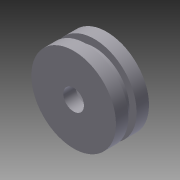
# Autodesk Inventor part: TU-005
Saved by Autodesk Inventor 2011 (Build 150229000, 229)
## iProperties
Created: 2008-06-13
Part Number: TU-005
Document SubType Name: Modeling
Designer: PN
Density: 2.71 g/cm^3
Material: Aluminum-6061
Description: Piston
Mass: 37.1113 g
Surface Area: 62.8633 cm^2
Volume: 13.6942 cm^3
Author: PN
Autodesk Inventor part; units mm, degrees
ref_plane "YZ Plane" through (0, 0, 0) normal (1, 0, 0) x (0, 1, 0)
ref_plane "XZ Plane" through (0, 0, 0) normal (0, 1, 0) x (-1, 0, 0)
ref_plane "XY Plane" through (0, 0, 0) normal (0, 0, 1) x (1, 0, 0)
sketch "Sketch1" plane through (0, 0, 0) normal (0, 0, 1) x (1, 0, 0)
  line L0 (20.5, 6) -> (20.5, 0)
  line L1 (20.5, 0) -> (5, 0)
  line L2 (5, 0) -> (5, 6)
  line L3 (5, 6) -> (13, 6)
  line L4 (13, 6) -> (13, 16)
  line L5 (13, 16) -> (20.5, 16)
  line L6 (20.5, 16) -> (20.5, 10)
  line L7 (20.5, 10) -> (17, 10)
  line L8 (17, 10) -> (17, 6)
  line L9 (17, 6) -> (20.5, 6)
  line L10 (0, 0) -> (0, 16) construction
  dimension "d0" = 10
  dimension "d1" = 26
  dimension "d2" = 34
  dimension "d3" = 41
  dimension "d4" = 6
  dimension "d5" = 10
  dimension "d6" = 16
  constraints: 22 end point, 2 collinear, 2 horizontal alignment, 1 horizontal, 1 perpendicular
  measures "d0" diameter of L2 L10
  measures "d1" diameter of L4 L10
  measures "d2" diameter of L8 L10
  measures "d3" diameter of L0 L10
  measures "d4" distance between parallel lines of L9 L1
  measures "d5" distance between parallel lines of L7 L1
  measures "d6" distance between parallel lines of L5 L1
revolve "Revolution1" add sketch "Sketch1" angle 360 about axis through (0, 0, 0) along (0, 1, 0)
body "Solid1"
